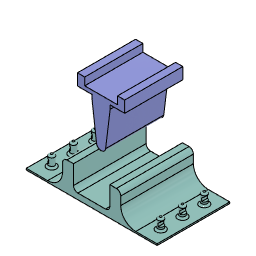
3D Printer Bend Test Jig_ (Autodesk Fusion 360 design; units mm, degrees)
Autodesk Fusion 360 part; units mm, degrees
sketch "Sketch1" plane through (0, 0, 0) normal (0, 1, 0) x (1, 0, 0)
  line L0 (-95, 75) -> (135, 75)
  line L1 (135, 75) -> (135, -115)
  line L2 (135, -115) -> (-95, -115)
  line L3 (-95, -115) -> (-95, 75)
  line L4 (0.9671, -13.4706) -> (33.9671, -13.4706)
  line L5 (33.9671, -13.4706) -> (33.9671, -19.4706)
  line L6 (33.9671, -19.4706) -> (0.9671, -19.4706)
  line L7 (0.9671, -19.4706) -> (0.9671, -13.4706)
  line L8 (-5, 35) -> (45, 35)
  line L9 (45, 35) -> (45, -65)
  line L10 (45, -65) -> (-5, -65)
  line L11 (-5, -65) -> (-5, 35)
  line L12 (-5, 35) -> (-20, 35)
  line L13 (-20, 35) -> (-20, -65)
  line L14 (-20, -65) -> (-5, -65)
  line L15 (-5, -65) -> (-5, 35)
  line L16 (45, 35) -> (60, 35)
  line L17 (60, 35) -> (60, -65)
  line L18 (60, -65) -> (45, -65)
  line L19 (45, -65) -> (45, 35)
  line L20 (-20, 35) -> (-70, 35)
  line L21 (-70, 35) -> (-70, 15)
  line L22 (-70, 15) -> (-20, 15)
  line L23 (-20, 15) -> (-20, 35)
  line L24 (60, 35) -> (110, 35)
  line L25 (110, 35) -> (110, 15)
  line L26 (110, 15) -> (60, 15)
  line L27 (60, 15) -> (60, 35)
  line L28 (60, -65) -> (110, -65)
  line L29 (110, -65) -> (110, -45)
  line L30 (110, -45) -> (60, -45)
  line L31 (60, -45) -> (60, -65)
  line L32 (-20, -65) -> (-70, -65)
  line L33 (-70, -65) -> (-70, -45)
  line L34 (-70, -45) -> (-20, -45)
  line L35 (-20, -45) -> (-20, -65)
  dimension "d1" = 230
  dimension "d2" = 190
  dimension "d3" = 33
  dimension "d4" = 6
  constraint horizontal L0
  constraint vertical L1
  constraint horizontal L2
  constraint vertical L3
  constraint horizontal L4
  constraint vertical L5
  constraint horizontal L6
  constraint vertical L7
  constraint horizontal L8
  constraint vertical L9
  constraint horizontal L10
  constraint vertical L11
  constraint horizontal L12
  constraint vertical L13
  constraint horizontal L14
  constraint vertical L15
  constraint horizontal L16
  constraint vertical L17
  constraint horizontal L18
  constraint vertical L19
  constraint horizontal L20
  constraint vertical L21
  constraint horizontal L22
  constraint vertical L23
  constraint horizontal L24
  constraint vertical L25
  constraint horizontal L26
  constraint vertical L27
  constraint horizontal L28
  constraint vertical L29
  constraint horizontal L30
  constraint vertical L31
  constraint horizontal L32
  constraint vertical L33
  constraint horizontal L34
  constraint vertical L35
  measures "d1" distance of L0.start L0.end
  measures "d2" distance of L0.start L2.end
  measures "d3" distance of L4.start L4.end
  measures "d4" distance of L4.start L6.end
extrude "Extrude1" add sketch "Sketch1" along normal blind 2 contours L8 L9 L10 L11 L15 L19 | L11 L12 L13 L14 L15 L23 L35 | L9 L16 L17 L18 L19 L27 L31 | L13 L20 L21 L22 L23 | L17 L24 L25 L26 L27 | L13 L32 L33 L34 L35 | L17 L28 L29 L30 L31 makes body 1
extrude "Extrude2" add sketch "Sketch1" along normal blind 8 separate body contours L4 L5 L6 L7 | L8 L9 L10 L11 L15 L19 makes body 2
extrude "Extrude3" add sketch "Sketch1" along normal blind 40 contours L11 L12 L13 L14 L15 L23 L35 | L9 L16 L17 L18 L19 L27 L31 bodies 1 2
fillet "Fillet1" radius 20.547 4 edges at (60, 2, -25) (60, 2, 55) (-20, 2, -25) (-20, 2, 55) on bodies 1
extrude "Extrude4" add 1 faces at (64.0367, 5.3701, -15) along direction (0, 0, 1) blind 64.644 on bodies 1 bodies 1
extrude "Extrude5" add 1 faces at (-24.0367, 5.3701, -15) along direction (0, 0, 1) blind 64.176 on bodies 1 bodies 1
sketch "Sketch2" plane through (0, 2, 0) normal (0, 1, 0) x (-1, 0, 0)
  line L0 (40.547, 65) -> (40.547, -35)
  line L1 (40.547, -35) -> (70, -35)
  line L2 (70, -35) -> (70, 65)
  line L3 (70, 65) -> (40.547, 65)
  circle A0 centre (55, -15) radius 4
  circle A1 centre (-95, -15) radius 4
  circle A2 centre (-95, 45) radius 4
  circle A3 centre (-95, 15) radius 4
  circle A4 centre (55, 15) radius 4
  circle A5 centre (55, 45) radius 4
  dimension "d17" = 8
  measures "d17" diameter of A0
extrude "Extrude6" add sketch "Sketch2" along normal blind 20 contours A0 | A1 | A2 | A3 | A4 | A5 bodies 1
sketch "Sketch3" plane through (0, 0, 65) normal (0, 0, 1) x (1, 0, 0)
  line L0 (-70, 0) -> (110, 0)
  line L1 (110, 0) -> (110, 2)
  line L2 (110, 2) -> (80.547, 2)
  arc A0 (60, 22.547) -> (80.547, 2) centre (80.547, 22.547) ccw
  line L3 (60, 22.547) -> (60, 40)
  line L4 (60, 40) -> (45, 40)
  line L5 (45, 40) -> (45, 8)
  line L6 (45, 8) -> (-5, 8)
  line L7 (-5, 8) -> (-5, 40)
  line L8 (-5, 40) -> (-20, 40)
  line L9 (-20, 40) -> (-20, 22.547)
  arc A1 (-40.547, 2) -> (-20, 22.547) centre (-40.547, 22.547) ccw
  line L10 (-40.547, 2) -> (-70, 2)
  line L11 (-70, 2) -> (-70, 0)
  line L12 (-60, 15) -> (-55.2735, 11.231)
  line L13 (-55.2735, 11.231) -> (-55.2735, 7)
  line L14 (-55.2735, 7) -> (-60, 7)
  line L15 (-60, 7) -> (-60, 15)
  line L16 (20, 8) -> (20, 20)
  line L17 (100, 15) -> (95.2735, 11.231)
  line L18 (100, 7) -> (100, 15)
  line L19 (95.2735, 7) -> (100, 7)
  line L20 (95.2735, 11.231) -> (95.2735, 7)
  constraint perpendicular L10 L13
  constraint perpendicular L13 L14
  constraint perpendicular L14 L15
  constraint midpoint L6 L16.start
  constraint perpendicular L6 L16
  constraint symmetric L12.start L16 L17.start
  constraint symmetric L12.end L16 L17.end
  constraint symmetric L13.end L16 L19.start
  constraint symmetric L14.end L16 L18.start
extrude "Extrude7" cut sketch "Sketch3" against normal blind 96.487 contours L12 L13 L14 L15 | L17 L18 L19 L20 bodies 1
extrude "Extrude8" cut 6 faces at (-53.7702, 22, -15.1987) (-55.9046, 22, 15.7214) (-54.5129, 22, 46.0682) (96.5708, 22, -15.9069) (94.8937, 22, 13.7588) (95.2967, 22, 43.8176) along direction (0, -1, 0) blind 5 on bodies 1 bodies 1
fillet "Fillet2" radius 2.487 12 edges at (-51.2707, 17, -13.5535) (-51.2707, 17, 16.4465) (-51.2707, 17, 46.4465) (98.7293, 17, -13.5535) (98.7293, 17, 16.4465) (98.7293, 17, 46.4465) (98.7293, 2, 46.4465) (98.7293, 2, 16.4465) (98.7293, 2, -13.5535) (-51.2707, 2, 46.4465) (-51.2707, 2, 16.4465) (-51.2707, 2, -13.5535) on bodies 1
fillet "Fillet3" radius 6.035 4 edges at (-20, 40, 15) (60, 40, 15) (45, 8, 15) (-5, 8, 15) on bodies 1
sketch "Sketch4" plane through (0, 0, 0) normal (0, 1, 0) x (1, 0, 0)
  line L0 (45, 205) -> (45, 184)
  line L1 (45, 184) -> (-30, 184)
  line L2 (-30, 184) -> (-30, 205)
  line L3 (30.0901, 205) -> (30.0901, 194.5)
  line L4 (30.0901, 194.5) -> (-15, 194.5)
  line L5 (-15, 194.5) -> (-15, 205)
  line L6 (7.5, 184) -> (-5, 184)
  line L7 (1.25, 134) -> (7.5, 134)
  line L8 (7.5, 134) -> (7.5, 184)
  line L9 (7.5, 134) -> (13.75, 134)
  line L10 (20, 184) -> (7.5, 184)
  line L11 (1.25, 134) -> (-5, 184)
  line L12 (13.75, 134) -> (20, 184)
  arc A0 (1.25, 134) -> (13.75, 134) centre (7.5, 134.7813) ccw
  line L13 (-30, 205) -> (-15, 205)
  line L14 (30.0901, 205) -> (45, 205)
  dimension "d28" = 75
  constraint horizontal L13
  constraint vertical L0
  constraint horizontal L1
  constraint vertical L2
  constraint vertical L3
  constraint horizontal L4
  constraint vertical L5
  constraint horizontal L6
  constraint horizontal L7
  constraint vertical L8
  constraint midpoint L1 L6.start
  constraint horizontal L9
  constraint horizontal L10
  constraint coincident L1 L10.start
  constraint tangent L12 A0
  constraint collinear L13 L14
  measures "d28" distance of L2.end L0.start
extrude "Extrude9" add sketch "Sketch4" along normal blind 80 separate body makes body 3
extrude "Extrude10" cut 1 faces at (45, 26.6667, -198) along direction (-1, 0, 0) blind 5 on bodies 3 bodies 3
extrude "Extrude11" cut 1 faces at (-30, 26.6667, -191) along direction (1, 0, 0) blind 5 on bodies 3 bodies 3
extrude "Extrude12" cut 2 faces at (-11.6667, 26.6667, -184) (33.3333, 53.3333, -184) along direction (0, 0, -1) blind 5.207 on bodies 3 bodies 3
move_body "Move1" bodies 3 to x (1, 0, 0) y (0, 1, 0) z (0, 0, 1) at (14.4975, 49.5966, 90.2277)
move_body "Move2" bodies 3 to x (1, 0, 0) y (0, 0, 1) z (0, -1, 0) at (0, 25.3244, -75.5412)
